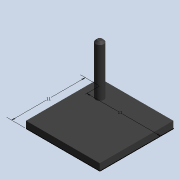
# Autodesk Inventor part: base
Saved by Autodesk Inventor 2020.2 (Build 242310000, 310)
## iProperties
Part Number: base
Material: Generic
Document SubType Name: Modeling
Designer: glg37
Appearance: Default
Author: glg37
Autodesk Inventor part; units mm, degrees
ref_plane "YZ Plane" through (0, 0, 0) normal (1, 0, 0) x (0, 1, 0)
ref_plane "XZ Plane" through (0, 0, 0) normal (0, 1, 0) x (-1, 0, 0)
ref_plane "XY Plane" through (0, 0, 0) normal (0, 0, 1) x (1, 0, 0)
sketch "Sketch1" plane through (0, 0, 0) normal (0, 1, 0) x (-1, 0, 0)
  line L0 (0, 0) -> (110, 0)
  line L1 (110, 0) -> (110, -110)
  line L2 (110, -110) -> (0, -110)
  line L3 (0, -110) -> (0, 0)
  dimension "d0" = 110
  dimension "d1" = 110
  constraints: 8 end point, 2 parallel, 1 horizontal, 1 perpendicular
  measures "d0" distance of L1.end L2.end
  measures "d1" distance of L0.end L1.end
extrude "Extrusion1" add sketch "Sketch1" along normal blind 10
sketch "Sketch2" plane through (0, 10, 0) normal (0, 1, 0) x (1, 0, 0)
  circle A0 centre (-85, 85) radius 6
  line L0 (-110, 110) -> (-110, 0) projected
  line L1 (0, 110) -> (-110, 110) projected
  line L2 (0, 0) -> (0, 110) projected
  line L3 (-110, 0) -> (0, 0) projected
  dimension "d11" = 12
  dimension "d12" = 25
  dimension "d13" = 25
  constraints: 1 centre point
  measures "d11" diameter of A0
  measures "d12" distance from line of L0 A0.centre
  measures "d13" distance from line of L1 A0.centre
extrude "Extrusion3" add sketch "Sketch2" along normal blind 75 contours A0
chamfer "Chamfer1" distance 3 angle 45 1 edges at (-91, 85, -85)
body "Solid1"
